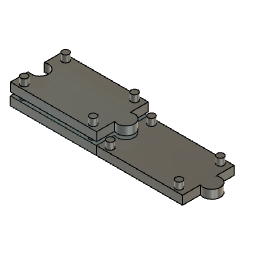
Module Simandre v1 (Autodesk Fusion 360 design; units mm, degrees)
Autodesk Fusion 360 part; units mm, degrees
sketch "Esquisse1" plane through (0, 0, 0) normal (0, 0, 1) x (1, 0, 0)
  line L0 (-50, 30) -> (0, 30)
  line L1 (0, 30) -> (0, 0)
  line L2 (0, 0) -> (-50, 0)
  line L3 (-50, 0) -> (-50, 30)
  constraint horizontal L0
  constraint vertical L1
  constraint horizontal L2
  constraint vertical L3
sketch "Esquisse2" plane through (0, 0, 0) normal (0, 0, 1) x (1, 0, 0)
  line L0 (-50, 15) -> (-48, 15)
  circle A0 centre (-48, 15) radius 5
  line L1 (0, 15) -> (2, 15)
  circle A1 centre (2, 15) radius 5
  constraint horizontal L0
  constraint coincident L0.end A0.centre
  constraint parallel L0 L1
  constraint coincident L1.end A1.centre
sketch "Esquisse3" plane through (0, 0, 0) normal (0, 0, 1) x (1, 0, 0)
sketch "Esquisse4" plane through (0, 0, 0) normal (0, 0, 1) x (1, 0, 0)
extrude "Extrusion1" add sketch "Esquisse1" along normal blind 5 makes body 1
extrude "Extrusion2" add sketch "Esquisse2" along normal blind 5 contours A1 bodies 1
sketch "Esquisse5" plane through (0, 0, 0) normal (0, 0, -1) x (1, 0, 0)
  line L0 (0, -10.4174) -> (0, 0)
  line L1 (0, 0) -> (-50, 0)
  line L2 (-50, 0) -> (-50, -30)
  line L3 (-50, -30) -> (0, -30)
  line L4 (0, -30) -> (0, -19.5826)
  arc A0 (0, -19.5826) -> (0, -10.4174) centre (2, -15) ccw
  line L5 (-50, -15) -> (-48, -15)
  circle A1 centre (-48, -15) radius 5
  constraint midpoint L2 L5.start
  constraint perpendicular L2 L5
  constraint coincident L5.end A1.centre
extrude "Extrusion3" cut sketch "Esquisse5" against normal blind 5 contours L2 A1 picked at (-45.35, -14.7648) bodies 1
sketch "Esquisse6" plane through (0, 0, 5) normal (0, 0, 1) x (-1, 0, 0)
  arc A0 (50, -10.4174) -> (50, -19.5826) centre (48, -15) ccw
  line L0 (50, -10.4174) -> (50, 0)
  line L1 (50, 0) -> (0, 0)
  line L2 (0, 0) -> (0, -10.4174)
  arc A1 (0, -10.4174) -> (0, -19.5826) centre (-2, -15) ccw
  line L3 (0, -19.5826) -> (0, -30)
  line L4 (0, -30) -> (50, -30)
  line L5 (50, -30) -> (50, -19.5826)
  circle A2 centre (45, -27) radius 2
  line L6 (45, -27) -> (50, -27)
  line L7 (0, -27) -> (5, -27)
  line L8 (5, -3) -> (5, 0)
  line L9 (45, -3) -> (45, 0)
  circle A3 centre (45, -3) radius 2
  circle A4 centre (5, -3) radius 2
  circle A5 centre (5, -27) radius 2
  constraint coincident A2.centre L6.start
  constraint coincident L5 L6.end
  constraint perpendicular L5 L6
  constraint coincident L3 L7.start
  constraint perpendicular L3 L7
  constraint coincident L1 L8.end
  constraint perpendicular L1 L8
  constraint coincident L1 L9.end
  constraint perpendicular L1 L9
  constraint coincident L9.start A3.centre
  constraint coincident L8.start A4.centre
  constraint coincident L7.end A5.centre
extrude "Extrusion4" add sketch "Esquisse6" along normal blind 2 contours A2 | A3 | A4 | A5 bodies 1
sketch "Esquisse7" plane through (0, 0, 0) normal (0, 0, -1) x (1, 0, 0)
  arc A0 (-50, -19.5826) -> (-50, -10.4174) centre (-48, -15) ccw
  line L0 (-50, -19.5826) -> (-50, -30)
  line L1 (-50, -30) -> (0, -30)
  line L2 (0, -30) -> (0, -19.5826)
  arc A1 (0, -19.5826) -> (0, -10.4174) centre (2, -15) ccw
  line L3 (0, -10.4174) -> (0, 0)
  line L4 (0, 0) -> (-50, 0)
  line L5 (-50, 0) -> (-50, -10.4174)
sketch "Esquisse8" plane through (0, 0, 5) normal (0, 0, 1) x (-1, 0, 0)
  circle A0 centre (45, -3) radius 2
  circle A1 centre (45, -27) radius 2
  circle A2 centre (5, -3) radius 2
  circle A3 centre (5, -27) radius 2
  arc A4 (50, -10.4174) -> (50, -19.5826) centre (48, -15) ccw
  line L0 (50, -10.4174) -> (50, 0)
  line L1 (50, 0) -> (0, 0)
  line L2 (0, 0) -> (0, -10.4174)
  arc A5 (0, -10.4174) -> (0, -19.5826) centre (-2, -15) ccw
  line L3 (0, -19.5826) -> (0, -30)
  line L4 (0, -30) -> (50, -30)
  line L5 (50, -30) -> (50, -19.5826)
sketch "Esquisse9" plane through (0, 0, 0) normal (0, 0, -1) x (1, 0, 0)
  line L0 (0, 0) -> (-5, 0)
  line L1 (-5, 0) -> (-5, -3)
  circle A0 centre (-5, -3) radius 2
  line L2 (0, -30) -> (-5, -30)
  line L3 (-5, -30) -> (-5, -27)
  circle A1 centre (-5, -27) radius 2
  line L4 (-50, 0) -> (-45, 0)
  line L5 (-45, 0) -> (-45, -3)
  circle A2 centre (-45, -3) radius 2
  line L6 (-50, -30) -> (-45, -30)
  line L7 (-45, -30) -> (-45, -27)
  circle A3 centre (-45, -27) radius 2
  constraint coincident L0.start origin
  constraint horizontal L0
  constraint perpendicular L0 L1
  constraint coincident L1.end A0.centre
  constraint horizontal L2
  constraint perpendicular L2 L3
  constraint coincident L3.end A1.centre
  constraint horizontal L4
  constraint perpendicular L4 L5
  constraint coincident L5.end A2.centre
  constraint horizontal L6
  constraint perpendicular L6 L7
  constraint coincident L7.end A3.centre
extrude "Extrusion5" cut sketch "Esquisse9" against normal blind 2 bodies 1
extrude "Extrusion6" add 4 faces at (-4.7564, 26.3794, 7) (-5.4887, 3.1251, 7) (-45.3535, 3.3078, 7) (-44.9285, 26.4788, 7) along direction (0, 0, 1) blind 2 on bodies 1 bodies 1
mirror "Symétrie miroir1" about plane through (0, 0, 0) normal (0, 1, 0) of bodies 1 makes body 2
move_body "Déplacer1" bodies 2 to x (1, 0, 0) y (0, 1, 0) z (0, 0, 1) at (0.4593, 30.6804, 7.3171)
move_body "Déplacer2" bodies 2 to x (1, 0, 0) y (0, 1, 0) z (0, 0, 1) at (0, -1, 0)
mirror "Symétrie miroir2" about plane through (-50, 30, 0) normal (0, 1, 0) of bodies 1 makes body 3
move_body "Déplacer3" bodies 3 to x (1, 0, 0) y (0, 1, 0) z (0, 0, 1) at (50, -30, 0)
